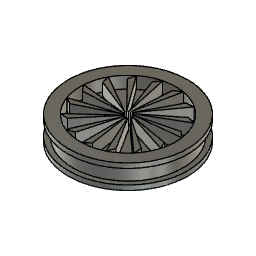
Wheel v1 (Autodesk Fusion 360 design; units mm, degrees)
Autodesk Fusion 360 part; units mm, degrees
sketch "Sketch1" plane through (0, 0, 0) normal (0, 0, 1) x (1, 0, 0)
  circle A0 centre (0, 0) radius 25
  constraint coincident A0.centre origin
extrude "Extrude1" add sketch "Sketch1" along normal blind 10
sketch "Sketch2" plane through (0, 0, 10) normal (0, 0, 1) x (-1, 0, 0)
  circle A0 centre (0, 0) radius 25
  circle A1 centre (0, 0) radius 1.5
  line L0 (0, 0) -> (1, 0)
  line L1 (1, 0) -> (1, -1.118)
  line L2 (1, 0) -> (1, 1.118)
  line L3 (1, -1.118) -> (1, 1.118)
  dimension "d3" = 3
  constraint coincident A0.centre A1.centre
  constraint horizontal L0
  constraint coincident A1 L1.end
  constraint perpendicular L0 L1
  constraint coincident A1 L2.end
  constraint perpendicular L0 L2
  measures "d3" diameter of A1
extrude "Extrude2" cut sketch "Sketch2" against normal blind 40 contours A1 L1 L2 L3 picked at (-0.6639, 0)
sketch "Sketch3" plane through (0, 0, 10) normal (0, 0, 1) x (-1, 0, 0)
  arc A0 (1, 1.118) -> (1, -1.118) centre (0, 0) ccw
  line L0 (1, 1.118) -> (1, -1.118)
  circle A1 centre (0, 0) radius 25
  circle A2 centre (0, 0) radius 20
  constraint concentric A0 A2
sketch "Sketch4" plane through (0, 0, 10) normal (0, 0, 1) x (-1, 0, 0)
  line L0 (0, 1.5) -> (7.5, 18.5)
  line L1 (7.5, 18.5) -> (4.5, 17.5)
  line L2 (4.5, 17.5) -> (0, 1.5)
  line L3 (-0.6101, 1.3703) -> (-0.673, 19.9511)
  line L4 (-3.0069, 17.8174) -> (-0.6101, 1.3703)
  line L5 (-0.673, 19.9511) -> (-3.0069, 17.8174)
  line L6 (-1.1147, 1.0037) -> (-8.7297, 17.9525)
  line L7 (-9.9939, 15.0539) -> (-1.1147, 1.0037)
  line L8 (-8.7297, 17.9525) -> (-9.9939, 15.0539)
  line L9 (-1.4266, 0.4635) -> (-15.2769, 12.8497)
  line L10 (-15.2529, 9.6876) -> (-1.4266, 0.4635)
  line L11 (-15.2769, 12.8497) -> (-15.2529, 9.6876)
  line L12 (-1.4918, -0.1568) -> (-19.1826, 5.5251)
  line L13 (-17.8745, 2.6461) -> (-1.4918, -0.1568)
  line L14 (-19.1826, 5.5251) -> (-17.8745, 2.6461)
  line L15 (-1.299, -0.75) -> (-19.7715, -2.7548)
  line L16 (-17.4054, -4.8529) -> (-1.299, -0.75)
  line L17 (-19.7715, -2.7548) -> (-17.4054, -4.8529)
  line L18 (-0.8817, -1.2135) -> (-16.9417, -10.5584)
  line L19 (-13.9268, -11.5128) -> (-0.8817, -1.2135)
  line L20 (-16.9417, -10.5584) -> (-13.9268, -11.5128)
  line L21 (-0.3119, -1.4672) -> (-11.1825, -16.5364)
  line L22 (-8.0401, -16.182) -> (-0.3119, -1.4672)
  line L23 (-11.1825, -16.5364) -> (-8.0401, -16.182)
  line L24 (0.3119, -1.4672) -> (-3.4897, -19.6551)
  line L25 (-0.7632, -18.0532) -> (0.3119, -1.4672)
  line L26 (-3.4897, -19.6551) -> (-0.7632, -18.0532)
  line L27 (0.8817, -1.2135) -> (4.8064, -19.3752)
  line L28 (6.6457, -16.8028) -> (0.8817, -1.2135)
  line L29 (4.8064, -19.3752) -> (6.6457, -16.8028)
  line L30 (1.299, -0.75) -> (12.2715, -15.7452)
  line L31 (12.9054, -12.6471) -> (1.299, -0.75)
  line L32 (12.2715, -15.7452) -> (12.9054, -12.6471)
  line L33 (1.4918, -0.1568) -> (17.6147, -9.3927)
  line L34 (16.9338, -6.3046) -> (1.4918, -0.1568)
  line L35 (17.6147, -9.3927) -> (16.9338, -6.3046)
  line L36 (1.4266, 0.4635) -> (19.9122, -1.4161)
  line L37 (18.0341, 1.128) -> (1.4266, 0.4635)
  line L38 (19.9122, -1.4161) -> (18.0341, 1.128)
  line L39 (1.1147, 1.0037) -> (18.7667, 6.8053)
  line L40 (16.0161, 8.3656) -> (1.1147, 1.0037)
  line L41 (18.7667, 6.8053) -> (16.0161, 8.3656)
  line L42 (0.6101, 1.3703) -> (14.3762, 13.8501)
  line L43 (11.2288, 14.1567) -> (0.6101, 1.3703)
  line L44 (14.3762, 13.8501) -> (11.2288, 14.1567)
  dimension "d7" = 360
extrude "Extrude3" cut sketch "Sketch3" against normal blind 5 contours A2
extrude "Extrude4" add sketch "Sketch4" against normal blind 5
sketch "Sketch5" plane through (0, 0, 0) normal (1, 0, 0) x (0, 1, 0)
  line L0 (-25, 2) -> (-25, 7)
  line L1 (-25, 7) -> (-20, 7)
  line L2 (-20, 2) -> (-25, 2)
  line L3 (-23, 7) -> (-23, 2)
  constraint vertical L0
  constraint perpendicular L0 L1
  constraint perpendicular L0 L2
  constraint coincident L1 L3.start
  constraint coincident L2 L3.end
  constraint perpendicular L2 L3
revolve "Revolve1" cut sketch "Sketch5" angle 360 about axis through (0, 0, 1.75) along (0, 0, 1)
sketch "Sketch6" plane through (0, 0, 0) normal (0, 0, -1) x (1, 0, 0)
  arc A0 (-1, -1.118) -> (-1, 1.118) centre (0, 0) ccw
  line L0 (-1, -1.118) -> (-1, 1.118)
  circle A1 centre (0, 0) radius 25
sketch "Sketch7" plane through (0, 0, 0) normal (0, 1, 0) x (1, 0, 0)
extrude "Extrude5" add 1 faces at (-1.7654, -23.5577, 2) along direction (0, 0, 1) blind 1
extrude "Extrude6" cut 1 faces at (-1.7654, -23.5577, 3) along direction (0, 0, -1) blind 1
extrude "Extrude7" cut 1 faces at (-1.7654, -23.5577, 7) along direction (0, 0, 1) blind 1
